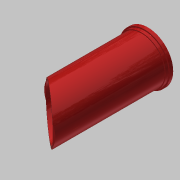
# Autodesk Inventor part: A1-19010-100-02 HCWI nozzle insert
Saved by Autodesk Inventor 2017.3 (Build 213257000, 257)
## iProperties
Created: 2014-07-18
Part Number: A1-19010-100-02 HCWI nozzle insert
Material: Iron, Cast
Document SubType Name: Modeling
Designer: Graeme_Van_Dongen
Density: 7.25 g/cm^3
Appearance: Light Red
Description: 30" HCWI NOZZLE, ASTM A532 CLASS III TYPE A, PF# 741278
Mass: 764103 g
Surface Area: 65145.1 cm^2
Volume: 105394 cm^3
Sheet Metal Width: 0.000 in
Sheet Metal Length: 0.000 in
Sheet Metal Area: 0.000 in^2
d0: 30.020 in
d1: 2.000 in
d2: 0.00 deg
d3: 28.520 in
d4: 3.750 in
d5: 0.00 deg
d6: 27.500 in
d7: 68.740 in
d8: 0.00 deg
d9: 25.000 in
d12: 0.00 deg
d13: 0.031 in
d16: 0.031 in
d17: 0.031 in
d18: 40.00 deg
d20: 0.00 deg
d24: 0.250 in
Author: Graeme_Van_Dongen
Autodesk Inventor part; units mm, degrees
ref_plane "YZ Plane" through (0, 0, 0) normal (1, 0, 0) x (0, 1, 0)
ref_plane "XZ Plane" through (0, 0, 0) normal (0, 1, 0) x (-1, 0, 0)
ref_plane "XY Plane" through (0, 0, 0) normal (0, 0, 1) x (1, 0, 0)
sketch "Sketch1" plane through (0, 0, 0) normal (0, 0, 1) x (1, 0, 0)
  circle A0 centre (0, 0) radius 381.254
  dimension "d0" = 762.508
  constraints: 1 centre point, 1 coincident
  measures "d0" diameter of A0
extrude "Extrusion1" add sketch "Sketch1" along normal blind 50.8
sketch "Sketch2" plane through (0, 0, 0) normal (0, 0, 1) x (1, 0, 0)
  circle A0 centre (0, 0) radius 362.204
  dimension "d3" = 724.408
  constraints: 1 centre point, 1 coincident
  measures "d3" diameter of A0
extrude "Extrusion2" add sketch "Sketch2" along normal blind 95.25
sketch "Sketch3" plane through (0, 0, 0) normal (0, 0, 1) x (1, 0, 0)
  circle A0 centre (0, 0) radius 349.25
  dimension "d6" = 698.5
  constraints: 1 centre point, 1 coincident
  measures "d6" diameter of A0
extrude "Extrusion3" add sketch "Sketch3" along normal blind 1746
sketch "Sketch4" plane through (0, 0, 1746) normal (0, 0, 1) x (1, 0, 0)
  circle A0 centre (-6.35, 0) radius 317.5
  point P0 (0, 0)
  dimension "d9" = 635
  dimension "d24" = 6.35
  constraints: 1 centre point, 1 horizontal alignment
  measures "d9" diameter of A0
  measures "d24" distance of point (0, 0) A0.centre
extrude "Extrusion4" cut sketch "Sketch4" against normal through all
chamfer "Chamfer1" distance 0.7937 angle 45 1 edges at (-381.254, 0, 50.8)
fillet "Fillet1" radius 0.7937 1 edges at (-362.204, 0, 50.8)
fillet "Fillet2" radius 0.7937 1 edges at (-349.25, 0, 95.25)
sketch "Sketch5" plane through (0, 0, 0) normal (0, 1, 0) x (-1, 0, 0)
  line L0 (-311.15, 1746) -> (323.85, 1746) projected
  line L1 (-311.15, 1746) -> (323.85, 1213.1717)
  line L2 (323.85, 1213.1717) -> (349.25, 1213.1717)
  line L3 (349.25, 1213.1717) -> (349.25, 1746)
  line L4 (349.25, 1746) -> (323.85, 1746)
  line L5 (349.25, 96.0438) -> (349.25, 1746) construction
  point P0 (0, 0)
  dimension "d18" = 40
  constraints: 8 end point, 2 perpendicular, 1 collinear, 1 parallel, 1 vertical alignment
  measures "d18" angle of L0 L1
extrude "Extrusion5" cut sketch "Sketch5" along normal through all both and the other way through all
equation "\"BendRadius\" = Thickness"
equation "\"BendReliefWidth\" = Thickness"
equation "\"BendReliefDepth\" = 0.5 * Thickness"
equation "\"CornerReliefSize\" = 4 * Thickness"
equation "\"MinimumRemnant\" = 2 * Thickness"
equation "\"TransitionRadius\" = BendRadius"
equation "\"JacobiRadiusSize\" = Thickness"
equation "\"GapSize\" = Thickness"
equation "\"Thickness\" = 3.048"
body "Solid1"
